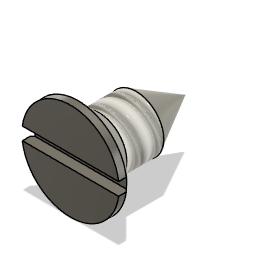
unplugged_Electrowizards_box (Autodesk Fusion 360 archive; units mm, degrees)
design "Countersunk Screw JIS B 1115 - ST2.2 x 4.5 - C Steel 4.6 Plain"
description: Countersunk Screw JIS B 1115 - ST2.2 x 4.5 - C
part number: CS JIS B 1115 - ST2.2 x 4.5 - C Steel 4.6 Plain
Autodesk Fusion 360 part; units mm, degrees
sketch "Sketch1" plane through (0, 0, 0) normal (0, 1, 0) x (1, 0, 0)
  line L0 (0, -2.2) -> (-1.9, -2.2)
  line L1 (-1.9, -2.2) -> (-1.9, -1.9)
  line L2 (-1.9, -1.9) -> (-1.1, -1.1)
  line L3 (-1.1, -1.1) -> (-1.1, 2.3)
  line L4 (-1.1, -1.1) -> (0, 0) construction
  line L5 (0, 2.3) -> (0, -2.2)
  line L6 (-1.1, 2.3) -> (0, 2.3)
  dimension "d5" = 45
  dimension "d9" = 2.2
  dimension "d11" = 3.8
  dimension "d71" = 1.1
  dimension "d85" = 4.5
  constraint perpendicular L0 L1
  constraint vertical L3
  constraint collinear L2 L4
  constraint perpendicular L0 L5
  constraint collinear L4.end L0.start L5.start
  constraint coincident L4.end L5
  constraint coincident origin L4
  constraint horizontal L0
  constraint horizontal L6
  measures "d5" angle of L4 L5
  measures "d71" distance of L0 L2.end
  measures "d85" distance of L0 L5.start
revolve "Revolve1" add sketch "Sketch1" angle 360 about axis through (0, 0, -2.3) along (0, 0, 1)
sketch "Sketch2" plane through (0, 0, 2.2) normal (0, 0, 1) x (1, 0, 0)
  circle A0 centre (0, 0) radius 1.9
  line L0 (1.75, 0) -> (22.5, 0)
  line L1 (1.9, 0.25) -> (-1.9, 0.25)
  line L2 (-1.9, 0.25) -> (-1.9, -0.25)
  line L3 (-1.9, -0.25) -> (1.9, -0.25)
  line L4 (1.9, 0.25) -> (1.9, -0.25)
  dimension "d86" = 0.5
  constraint perpendicular L1 L2
  constraint tangent A0 L4
  constraint tangent A0 L2
  constraint perpendicular L1 L4
  constraint symmetric L0 L1 L3
  constraint perpendicular L2 L3
  constraint coincident L3.end L4.end
  measures "d86" distance of L1 L2.end
extrude "Extrude2" cut sketch "Sketch2" against normal blind 0.4 contours A0 L1 L3
thread "Thread1" "Metric Forming Screw Threads 2.2 ST2.2x0.8 6g" major diameter 2.17 minor diameter 1.575 pitch 0.8 angle 60 resizes the face on face at (-1.0986, 0.0548, -0.0333)
sketch "Sketch6" plane through (0, 0, 0) normal (0, 1, 0) x (1, 0, 0)
  line L0 (-1.122, 2.3) -> (-1.122, 0.3)
  line L1 (-1.122, 0.3) -> (0, 2.3)
  line L2 (0, 2.3) -> (0, -2.2)
  line L3 (-1.122, 2.3) -> (0, 2.3)
  dimension "d87" = 1.122
  dimension "d88" = 2
  constraint coincident L1.end L2.start
  constraint perpendicular L2 L3
  constraint coincident L1.end L3
  constraint perpendicular L0 L3
  measures "d87" distance of L0 L1.end
  measures "d88" distance of L0.end L3
revolve "Revolve3" cut sketch "Sketch6" angle 360 about axis through (0, 0, 1.75) along (0, 0, 1)
equation "d5 = adsk_headang * 0.5"
equation "d9 = adsk_nomdia"
equation "d11 = adsk_headdia"
equation "adsk_nomlen = 4.50 mm"
equation "adsk_headh = 1.10 mm"
equation "adsk_headdia = 3.80 mm"
equation "adsk_nomdia = 2.20 mm"
equation "adsk_headang = 90.00 deg"
equation "adsk_slotw = 0.50 mm"
equation "adsk_slotdepth = 0.40 mm"
equation "d67 = -adsk_slotdepth"
equation "adsk_startlen = 2.00 mm"
equation "d71 = adsk_headh"
equation "d78 = ( adsk_nomdia / 2 ) * tan(90 deg - adsk_headang / 2) + adsk_headh"
equation "d85 = adsk_nomlen"
equation "d86 = adsk_slotw"
equation "d87 = adsk_nomdia * 0.51"
equation "d88 = adsk_startlen"
